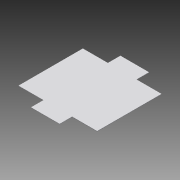
# Autodesk Inventor part: Aluminum Board
Saved by Autodesk Inventor 2014 SP1 (Build 180222100, 222)
## iProperties
Created: 2014-01-18
Part Number: Aluminum Board
Material: Generic
Document SubType Name: Modeling
Designer: Paul
Density: 1 g/cm^3
Appearance: Aluminum - Polished
Author: Paul
Autodesk Inventor part; units mm, degrees
ref_plane "YZ Plane" through (0, 0, 0) normal (1, 0, 0) x (0, 1, 0)
ref_plane "XZ Plane" through (0, 0, 0) normal (0, 1, 0) x (-1, 0, 0)
ref_plane "XY Plane" through (0, 0, 0) normal (0, 0, 1) x (1, 0, 0)
sketch "Sketch1" plane through (0, 0, 0) normal (0, 1, 0) x (-1, 0, 0)
  line L0 (0, 0) -> (0, 88.9)
  line L1 (0, 88.9) -> (-177.8, 88.9)
  line L2 (-177.8, 88.9) -> (-177.8, 546.1)
  line L3 (-177.8, 546.1) -> (0, 546.1)
  line L4 (0, 546.1) -> (0, 635)
  line L5 (0, 635) -> (203.2, 635)
  line L6 (203.2, 635) -> (203.2, 546.1)
  line L7 (203.2, 546.1) -> (381, 546.1)
  line L8 (381, 546.1) -> (381, 88.9)
  line L9 (381, 88.9) -> (203.2, 88.9)
  line L10 (203.2, 88.9) -> (203.2, 0)
  line L11 (203.2, 0) -> (0, 0)
  dimension "d0" = 88.9
  dimension "d1" = 177.8
  dimension "d2" = 88.9
  dimension "d3" = 177.8
  dimension "d4" = 177.8
  dimension "d5" = 88.9
  dimension "d6" = 177.8
  dimension "d7" = 88.9
  dimension "d8" = 558.8
  dimension "d9" = 635
  constraints: 24 end point, 8 parallel, 2 collinear, 1 perpendicular, 1 vertical
  measures "d0" distance of L9.end L10.end
  measures "d1" distance of L8.end L9.end
  measures "d2" distance of L5.end L6.end
  measures "d3" distance of L6.end L7.end
  measures "d4" distance of L2.end L3.end
  measures "d5" distance of L3.end L4.end
  measures "d6" distance of L0.end L1.end
  measures "d7" distance of L0.start L0.end
  measures "d8" distance between parallel lines of L8 L2
  measures "d9" distance between parallel lines of L11 L5
extrude "Extrusion1" add sketch "Sketch1" along normal blind 3.175
body "Solid1"
